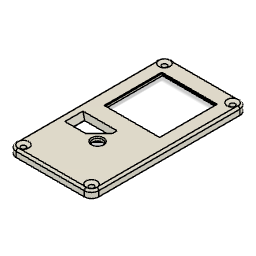
Marauder-Mini-Assembly (Autodesk Fusion 360 archive; units mm, degrees)
design "Marauder-Mini_Top_cutout"
Autodesk Fusion 360 part; units mm, degrees
sketch "Skizze1" plane through (0, 0, 0) normal (0, 1, 0) x (1, 0, 0)
  line L0 (1.75, 0) -> (22.5, 0)
  line L1 (0, -1.75) -> (0, -22.5)
  line L2 (-16.61, 36.93) -> (16.61, 36.93)
  line L3 (19.15, 34.39) -> (19.15, -34.39)
  line L4 (16.61, -36.93) -> (-16.61, -36.93)
  line L5 (-19.15, -34.39) -> (-19.15, 34.39)
  arc A0 (-16.61, 36.93) -> (-19.15, 34.39) centre (-16.61, 34.39) ccw
  arc A1 (19.15, 34.39) -> (16.61, 36.93) centre (16.61, 34.39) ccw
  arc A2 (16.61, -36.93) -> (19.15, -34.39) centre (16.61, -34.39) ccw
  arc A3 (-19.15, -34.39) -> (-16.61, -36.93) centre (-16.61, -34.39) ccw
  arc A4 (20.15, 34.39) -> (16.61, 37.93) centre (16.61, 34.39) ccw
  line L6 (-16.61, 37.93) -> (16.61, 37.93)
  arc A5 (-16.61, 37.93) -> (-20.15, 34.39) centre (-16.61, 34.39) ccw
  line L7 (-20.15, -34.39) -> (-20.15, 34.39)
  arc A6 (-20.15, -34.39) -> (-16.61, -37.93) centre (-16.61, -34.39) ccw
  line L8 (16.61, -37.93) -> (-16.61, -37.93)
  arc A7 (16.61, -37.93) -> (20.15, -34.39) centre (16.61, -34.39) ccw
  line L9 (20.15, 34.39) -> (20.15, -34.39)
  line L10 (-15.5, 32.25) -> (15.5, 32.25)
  line L11 (15.5, 32.25) -> (15.5, -4.75)
  line L12 (15.5, -4.75) -> (-15.5, -4.75)
  line L13 (-15.5, -4.75) -> (-15.5, 32.25)
  circle A8 centre (-16.61, 34.39) radius 1.2
  circle A9 centre (16.61, 34.39) radius 1.2
  circle A10 centre (-16.61, -34.39) radius 1.2
  circle A11 centre (16.61, -34.39) radius 1.2
  line L14 (-6.35, -27.43) -> (6.35, -27.43)
  line L15 (6.35, -27.43) -> (6.35, -35.43)
  line L16 (6.35, -35.43) -> (-6.35, -35.43)
  line L17 (-6.35, -35.43) -> (-6.35, -27.43)
  line L18 (-1.864, -10.43) -> (-4.5, -13.066)
  line L19 (-4.5, -13.066) -> (-4.5, -16.794)
  line L20 (-4.5, -16.794) -> (-1.864, -19.43)
  line L21 (-1.864, -19.43) -> (1.864, -19.43)
  line L22 (1.864, -19.43) -> (4.5, -16.794)
  line L23 (4.5, -16.794) -> (4.5, -13.066)
  line L24 (4.5, -13.066) -> (1.864, -10.43)
  line L25 (1.864, -10.43) -> (-1.864, -10.43)
  line L26 (0.5, -5.65) -> (15.5, -5.65)
  line L27 (15.5, -5.65) -> (15.5, -13.65)
  line L28 (15.5, -13.65) -> (6.5, -13.65)
  line L29 (6.5, -13.65) -> (0.5, -7.65)
  line L30 (0.5, -7.65) -> (0.5, -5.65)
  point P0 (-19.15, 36.93)
  point P1 (19.15, 36.93)
  point P2 (-19.15, -36.93)
  point P3 (0, -14.93)
  point P4 (0, -4.75)
  dimension "d1" = 73.86
  dimension "d2" = 38.3
  dimension "d3" = 2.54
  dimension "d4" = -1
  dimension "d5" = 31
  dimension "d7" = 2.4
  dimension "d8" = 37
  dimension "d9" = 8
  dimension "d10" = 12.7
  dimension "d11" = 1.5
  dimension "d12" = 22
  dimension "d24" = 4.5
  dimension "d27" = 8
  dimension "d28" = 15
  dimension "d30" = 2
  dimension "d47" = 5.65
  dimension "d48" = 4.75
  constraint horizontal L2
  constraint vertical L3
  constraint horizontal L4
  constraint vertical L5
  constraint symmetric L0 L2 L4
  constraint symmetric L1 L3 L5
  constraint coincident P0 L2
  constraint coincident P0 L5
  constraint tangent L2 A0
  constraint tangent L5 A0
  constraint coincident P1 L2
  constraint coincident P1 L3
  constraint tangent L2 A1
  constraint tangent L3 A1
  constraint equal A0 A1
  constraint tangent L3 A2
  constraint tangent L4 A2
  constraint equal A0 A2
  constraint coincident P2 L4
  constraint coincident P2 L5
  constraint tangent L4 A3
  constraint tangent L5 A3
  constraint equal A0 A3
  constraint horizontal L10
  constraint vertical L11
  constraint horizontal L12
  constraint vertical L13
  constraint symmetric L1 L11 L13
  constraint concentric A0 A8
  constraint concentric A1 A9
  constraint concentric A3 A10
  constraint concentric A2 A11
  constraint equal A10 A11
  constraint equal A9 A11
  constraint equal A8 A9
  constraint horizontal L14
  constraint vertical L15
  constraint horizontal L16
  constraint vertical L17
  constraint symmetric L1 L15 L17
  constraint horizontal L25
  constraint midpoint L12 P4
  constraint vertical P3 P4
  constraint horizontal L26
  constraint perpendicular L26 L27
  constraint perpendicular L27 L28
  constraint vertical L30
  constraint parallel L24 L29
  constraint collinear L11 L27
  constraint coincident L28.end L29.start
  measures "d1" distance of P0 P2
  measures "d2" distance of P0 P1
  measures "d3" radius of A0
  measures "d5" distance of L10.start L10.end
  measures "d7" diameter of A8
  measures "d8" distance of L10.end L11.end
  measures "d9" distance of L14.end L15.end
  measures "d10" distance of L15.end L16.end
  measures "d11" distance of L4 L16
  measures "d12" distance of L4 P3
  measures "d24" distance of P3 L25
  measures "d27" distance of L26.end L27.end
  measures "d28" distance of L26.start L26.end
  measures "d30" distance of L26.start L29.end
  measures "d47" distance of origin L26
  measures "d48" distance of origin L12
extrude "Extrusion1" add sketch "Skizze1" along normal blind 2 contours L2 L3 L4 L5 A0 A1 A2 A3 | A4 L6 A5 L7 A6 L8 A7 L9 makes body 1
sketch "Skizze2" plane through (0, 2, 0) normal (0, 1, 0) x (-1, 0, 0)
  circle A0 centre (16.61, -34.39) radius 1.2
  line L0 (-6.35, 35.43) -> (6.35, 35.43)
  line L1 (6.35, 35.43) -> (6.35, 27.43)
  line L2 (6.35, 27.43) -> (-6.35, 27.43)
  line L3 (-6.35, 27.43) -> (-6.35, 35.43)
  circle A1 centre (-16.61, 34.39) radius 1.2
  circle A2 centre (-16.61, -34.39) radius 1.2
  circle A3 centre (16.61, 34.39) radius 1.2
  line L4 (-15.5, 4.75) -> (15.5, 4.75)
  line L5 (15.5, 4.75) -> (15.5, -32.25)
  line L6 (15.5, -32.25) -> (-15.5, -32.25)
  line L7 (-15.5, -32.25) -> (-15.5, 4.75)
  arc A4 (16.61, -37.93) -> (20.15, -34.39) centre (16.61, -34.39) ccw
  line L8 (20.15, -34.39) -> (20.15, 34.39)
  arc A5 (20.15, 34.39) -> (16.61, 37.93) centre (16.61, 34.39) ccw
  line L9 (16.61, 37.93) -> (-16.61, 37.93)
  arc A6 (-16.61, 37.93) -> (-20.15, 34.39) centre (-16.61, 34.39) ccw
  line L10 (-20.15, 34.39) -> (-20.15, -34.39)
  arc A7 (-20.15, -34.39) -> (-16.61, -37.93) centre (-16.61, -34.39) ccw
  line L11 (-16.61, -37.93) -> (16.61, -37.93)
  circle A8 centre (0, 14.83) radius 2.5
  line L12 (1.864, 10.43) -> (-1.864, 10.43)
  line L13 (-1.864, 10.43) -> (-4.5, 13.066)
  line L14 (-4.5, 13.066) -> (-4.5, 16.794)
  line L15 (-4.5, 16.794) -> (-1.864, 19.43)
  line L16 (-1.864, 19.43) -> (1.864, 19.43)
  line L17 (1.864, 19.43) -> (4.5, 16.794)
  line L18 (4.5, 16.794) -> (4.5, 13.066)
  line L19 (4.5, 13.066) -> (1.864, 10.43)
  line L20 (-6.5, 13.65) -> (-0.5, 7.65)
  line L21 (-0.5, 7.65) -> (-0.5, 5.65)
  line L22 (-0.5, 5.65) -> (-15.5, 5.65)
  line L23 (-15.5, 5.65) -> (-15.5, 13.65)
  line L24 (-15.5, 13.65) -> (-6.5, 13.65)
  dimension "d16" = 5
  measures "d16" diameter of A8
extrude "Extrusion2" add sketch "Skizze2" along normal blind 1 contours L0 L1 L2 L3 | A4 L8 A5 L9 A6 L10 A7 L11 | L12 L13 L14 L15 L16 L17 L18 L19 bodies 1
chamfer "Fase4" distance 0.5 distance2 1 8 edges at (4.5, 2, 14.93) (3.182, 2, 18.112) (0, 2, 19.43) (-3.182, 2, 18.112) (-4.5, 2, 14.93) (-3.182, 2, 11.748) (3.182, 2, 11.748) (0, 2, 10.43) measured on face at (0.0623, 2, 18.7277) measured on face at (0.0623, 2, 18.7277) measured on face at (0.0623, 2, 18.7277) measured on face at (0.0623, 2, 18.7277) measured on face at (0.0623, 2, 18.7277) measured on face at (0.0623, 2, 18.7277) measured on face at (0.0623, 2, 18.7277) measured on face at (0.0623, 2, 18.7277) on bodies 1
sketch "Skizze3" plane through (0, 3, 0) normal (0, 1, 0) x (-1, 0, 0)
  circle A0 centre (0, 14.83) radius 2.5
  circle A1 centre (-16.61, -34.39) radius 1.2
  circle A2 centre (16.61, -34.39) radius 1.2
  line L0 (15.5, -32.25) -> (-15.5, -32.25)
  line L1 (-15.5, -32.25) -> (-15.5, 4.75)
  line L2 (-15.5, 4.75) -> (15.5, 4.75)
  line L3 (15.5, 4.75) -> (15.5, -32.25)
  circle A3 centre (-16.61, 34.39) radius 1.2
  line L4 (-15.5, 5.65) -> (-15.5, 13.65)
  line L5 (-15.5, 13.65) -> (-6.5, 13.65)
  line L6 (-6.5, 13.65) -> (-0.5, 7.65)
  line L7 (-0.5, 7.65) -> (-0.5, 5.65)
  line L8 (-0.5, 5.65) -> (-15.5, 5.65)
  circle A4 centre (16.61, 34.39) radius 1.2
  line L9 (-16.61, -37.93) -> (16.61, -37.93)
  arc A5 (16.61, -37.93) -> (20.15, -34.39) centre (16.61, -34.39) ccw
  line L10 (20.15, -34.39) -> (20.15, 34.39)
  arc A6 (20.15, 34.39) -> (16.61, 37.93) centre (16.61, 34.39) ccw
  line L11 (16.61, 37.93) -> (-16.61, 37.93)
  arc A7 (-16.61, 37.93) -> (-20.15, 34.39) centre (-16.61, 34.39) ccw
  line L12 (-20.15, 34.39) -> (-20.15, -34.39)
  arc A8 (-20.15, -34.39) -> (-16.61, -37.93) centre (-16.61, -34.39) ccw
  line L13 (0, 1.75) -> (0, 22.5)
  line L14 (13.5, -29.93) -> (-13.5, -29.93)
  line L15 (-13.5, -29.93) -> (-13.5, -1.93)
  line L16 (-13.5, -1.93) -> (13.5, -1.93)
  line L17 (13.5, -1.93) -> (13.5, -29.93)
  dimension "d33" = 27
  dimension "d49" = 28
  dimension "d50" = 8
  constraint horizontal L14
  constraint vertical L15
  constraint horizontal L16
  constraint vertical L17
  constraint symmetric L13 L15 L17
  measures "d33" distance of L15 L17
  measures "d49" distance of L14 L16
  measures "d50" distance of L9 L14
extrude "Extrusion3" add sketch "Skizze3" along normal blind 0.6 contours L0 L1 L2 L3 | L9 A5 L10 A6 L11 A7 L12 A8 bodies 1
fillet "Abrundung2" radius 1 8 edges at (0, 3.6, 37.93) (19.1132, 3.6, 36.8932) (20.15, 3.6, 0) (19.1132, 3.6, -36.8932) (0, 3.6, -37.93) (-19.1132, 3.6, -36.8932) (-20.15, 3.6, 0) (-19.1132, 3.6, 36.8932) on bodies 1
chamfer "Fase5" distance 1.5 distance2 1 4 edges at (-15.4912, 3.6, -33.9561) (17.7288, 3.6, -33.9561) (17.7288, 3.6, 34.8239) (-15.4912, 3.6, 34.8239) measured on face at (0, 3.6, 28.5841) measured on face at (0, 3.6, 28.5841) measured on face at (0, 3.6, 28.5841) measured on face at (0, 3.6, 28.5841) on bodies 1
chamfer "Fase6" distance 0.5 distance2 0.5 1 edges at (2.3308, 3.6, 15.734) measured on face at (-0.0585, 3.6, 28.4655) on bodies 1
chamfer "Fase6" distance 2 angle 45 4 edges at (0, 2, 27.43) (-6.35, 2, 31.43) (0, 2, 35.43) (6.35, 2, 31.43) on bodies 1
chamfer "Fase7" distance 0.8 distance2 3.5 4 edges at (0.5, 3.6, 6.65) (3.5, 3.6, 10.65) (11, 3.6, 13.65) (15.5, 3.6, 9.65) measured on face at (-0.071, 3.6, 28.6317) measured on face at (-0.071, 3.6, 28.6317) measured on face at (-0.071, 3.6, 28.6317) measured on face at (-0.071, 3.6, 28.6317) on bodies 1
mirror "Spiegeln1" about plane through (20.15, 3, 34.39) normal (1, 0, 0) of bodies 1 makes body 2
hidden bodies 1
equation "d5 = 30.1 mm + 0.9 mm"
named bodies: "MarauderMini-Top"

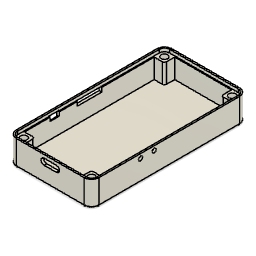
design "Marauder-Mini_Bottom"
Autodesk Fusion 360 part; units mm, degrees
sketch "Skizze1" plane through (0, 0, 0) normal (0, 1, 0) x (1, 0, 0)
  line L0 (-16.51, 36.83) -> (16.51, 36.83)
  line L1 (19.05, 34.29) -> (19.05, -34.29)
  line L2 (16.51, -36.83) -> (-16.51, -36.83)
  line L3 (-19.05, -34.29) -> (-19.05, 34.29)
  line L4 (1.75, 0) -> (22.5, 0)
  line L5 (0, -1.75) -> (0, -22.5)
  arc A0 (-16.51, 36.83) -> (-19.05, 34.29) centre (-16.51, 34.29) ccw
  arc A1 (19.05, 34.29) -> (16.51, 36.83) centre (16.51, 34.29) ccw
  arc A2 (16.51, -36.83) -> (19.05, -34.29) centre (16.51, -34.29) ccw
  arc A3 (-19.05, -34.29) -> (-16.51, -36.83) centre (-16.51, -34.29) ccw
  arc A4 (20.15, 34.29) -> (16.51, 37.93) centre (16.51, 34.29) ccw
  line L6 (-16.51, 37.93) -> (16.51, 37.93)
  arc A5 (-16.51, 37.93) -> (-20.15, 34.29) centre (-16.51, 34.29) ccw
  line L7 (-20.15, -34.29) -> (-20.15, 34.29)
  arc A6 (-20.15, -34.29) -> (-16.51, -37.93) centre (-16.51, -34.29) ccw
  line L8 (16.51, -37.93) -> (-16.51, -37.93)
  arc A7 (16.51, -37.93) -> (20.15, -34.29) centre (16.51, -34.29) ccw
  line L9 (20.15, 34.29) -> (20.15, -34.29)
  point P0 (-19.05, 36.83)
  point P1 (19.05, 36.83)
  point P2 (-19.05, -36.83)
  dimension "d1" = 73.66
  dimension "d2" = 38.1
  dimension "d3" = 2.54
  dimension "d4" = -1.1
  constraint horizontal L0
  constraint vertical L1
  constraint horizontal L2
  constraint vertical L3
  constraint symmetric L0 L2 L4
  constraint symmetric L1 L3 L5
  constraint coincident P0 L0
  constraint coincident P0 L3
  constraint tangent L0 A0
  constraint tangent L3 A0
  constraint coincident P1 L0
  constraint coincident P1 L1
  constraint tangent L0 A1
  constraint tangent L1 A1
  constraint equal A0 A1
  constraint tangent L1 A2
  constraint tangent L2 A2
  constraint equal A0 A2
  constraint coincident P2 L2
  constraint coincident P2 L3
  constraint tangent L2 A3
  constraint tangent L3 A3
  constraint equal A0 A3
  measures "d1" distance of P0 P2
  measures "d2" distance of P0 P1
  measures "d3" radius of A0
extrude "Extrusion1" add sketch "Skizze1" along normal blind 1.5 contours L0 L1 L2 L3 A0 A1 A2 A3 | A4 L6 A5 L7 A6 L8 A7 L9
sketch "Skizze2" plane through (0, 1.5, 0) normal (0, 1, 0) x (-1, 0, 0)
  arc A0 (16.51, -37.93) -> (20.15, -34.29) centre (16.51, -34.29) ccw
  line L0 (20.15, -34.29) -> (20.15, 34.29)
  arc A1 (20.15, 34.29) -> (16.51, 37.93) centre (16.51, 34.29) ccw
  line L1 (16.51, 37.93) -> (-16.51, 37.93)
  arc A2 (-16.51, 37.93) -> (-20.15, 34.29) centre (-16.51, 34.29) ccw
  line L2 (-20.15, 34.29) -> (-20.15, -34.29)
  arc A3 (-20.15, -34.29) -> (-16.51, -37.93) centre (-16.51, -34.29) ccw
  line L3 (-16.51, -37.93) -> (16.51, -37.93)
  line L4 (18.85, -34.29) -> (18.85, 34.29)
  arc A4 (18.85, 34.29) -> (16.51, 36.63) centre (16.51, 34.29) ccw
  line L5 (16.51, 36.63) -> (-16.51, 36.63)
  arc A5 (-16.51, 36.63) -> (-18.85, 34.29) centre (-16.51, 34.29) ccw
  line L6 (-18.85, 34.29) -> (-18.85, -34.29)
  arc A6 (-18.85, -34.29) -> (-16.51, -36.63) centre (-16.51, -34.29) ccw
  line L7 (-16.51, -36.63) -> (16.51, -36.63)
  arc A7 (16.51, -36.63) -> (18.85, -34.29) centre (16.51, -34.29) ccw
  circle A8 centre (16.51, -34.29) radius 1.65
  circle A9 centre (-16.51, -34.29) radius 1.65
  circle A10 centre (-16.51, 34.29) radius 1.65
  circle A11 centre (16.51, 34.29) radius 1.65
  line L8 (13.85, -36.63) -> (13.85, -32.63)
  line L9 (14.85, -31.63) -> (18.85, -31.63)
  line L10 (-13.85, -36.63) -> (-13.85, -32.63)
  line L11 (-14.85, -31.63) -> (-18.85, -31.63)
  line L12 (18.85, 31.63) -> (14.85, 31.63)
  line L13 (13.85, 32.63) -> (13.85, 36.63)
  line L14 (-13.85, 36.63) -> (-13.85, 32.63)
  line L15 (-14.85, 31.63) -> (-18.85, 31.63)
  line L16 (-1.75, 0) -> (-22.5, 0)
  line L17 (0, 1.75) -> (0, 22.5)
  arc A12 (14.85, -31.63) -> (13.85, -32.63) centre (14.85, -32.63) ccw
  arc A13 (-13.85, -32.63) -> (-14.85, -31.63) centre (-14.85, -32.63) ccw
  arc A14 (13.85, 32.63) -> (14.85, 31.63) centre (14.85, 32.63) ccw
  arc A15 (-14.85, 31.63) -> (-13.85, 32.63) centre (-14.85, 32.63) ccw
  point P0 (13.85, -31.63)
  dimension "d7" = -1.3
  dimension "d8" = 3.3
  dimension "d9" = 5
  dimension "d10" = 5
  dimension "d11" = 1
  constraint concentric A0 A8
  constraint concentric A3 A9
  constraint concentric A2 A10
  constraint concentric A1 A11
  constraint equal A8 A9
  constraint equal A9 A10
  constraint equal A10 A11
  constraint coincident L7 L8.start
  constraint perpendicular L7 L8
  constraint coincident L4 L9.end
  constraint perpendicular L4 L9
  constraint coincident L7 L10.start
  constraint perpendicular L7 L10
  constraint perpendicular L10 L11
  constraint coincident L4 L12.start
  constraint perpendicular L4 L12
  constraint coincident L5 L13.end
  constraint perpendicular L5 L13
  constraint coincident L5 L14.start
  constraint perpendicular L5 L14
  constraint perpendicular L14 L15
  constraint collinear L9 L11
  constraint collinear L8 L13
  constraint collinear L12 L15
  constraint collinear L10 L14
  constraint symmetric L9 L12 L16
  constraint symmetric L8 L10 L17
  constraint coincident P0 L8
  constraint coincident P0 L9
  constraint tangent L8 A12
  constraint tangent L9 A12
  constraint tangent L10 A13
  constraint tangent L11 A13
  constraint equal A12 A13
  constraint tangent L12 A14
  constraint tangent L13 A14
  constraint equal A12 A14
  constraint tangent L14 A15
  constraint tangent L15 A15
  constraint equal A12 A15
  constraint coincident L6 L11.end
  constraint coincident L6 L15.end
  measures "d8" diameter of A8
  measures "d9" distance of L8.start P0
  measures "d10" distance of P0 L9.end
  measures "d11" radius of A12
extrude "Extrusion2" add sketch "Skizze2" along normal blind 9.5 contours A0 L0 A1 L1 A2 L2 A3 L3 | L4 L7 A7 L8 L9 A12 | L4 A4 L5 L12 L13 A14 | L6 A6 L7 L10 L11 A13 | L5 A5 L6 L14 L15 A15
fillet "Abrundung1" radius 1 8 edges at (-19.0839, 0, -36.8639) (0, 0, -37.93) (19.0839, 0, -36.8639) (20.15, 0, 0) (19.0839, 0, 36.8639) (0, 0, 37.93) (-19.0839, 0, 36.8639) (-20.15, 0, 0)
sketch "Skizze3" plane through (0, 0, 37.93) normal (0, 0, 1) x (1, 0, 0)
  line L0 (-16.51, 1) -> (16.51, 1)
  line L1 (16.51, 1) -> (16.51, 11)
  line L2 (16.51, 11) -> (-16.51, 11)
  line L3 (-16.51, 11) -> (-16.51, 1)
  line L4 (-4.5, 11) -> (4.5, 11)
  line L5 (4.5, 11) -> (4.5, 8)
  line L6 (4.5, 8) -> (-4.5, 8)
  line L7 (-4.5, 8) -> (-4.5, 11)
  line L8 (0, 1.75) -> (0, 22.5)
  dimension "d16" = 9
  dimension "d17" = 3
  constraint horizontal L4
  constraint vertical L5
  constraint horizontal L6
  constraint vertical L7
  constraint coincident L2 L4.start
  constraint symmetric L5 L7 L8
  measures "d16" distance of L5.end L6.end
  measures "d17" distance of L4.start L6.end
extrude "Extrusion3" cut sketch "Skizze3" against normal blind 2 contours L2 L4 L6 L7 L8 | L2 L4 L5 L6 L8
sketch "Skizze4" plane through (-20.15, 0, 0) normal (-1, 0, 0) x (0, 0, 1)
  line L0 (-34.29, 1) -> (34.29, 1)
  line L1 (34.29, 11) -> (-34.29, 11)
  line L2 (-34.29, 11) -> (-34.29, 1)
  line L3 (14.63, 11) -> (19.13, 11)
  line L4 (19.13, 11) -> (19.13, 9.2)
  line L5 (19.13, 9.2) -> (14.63, 9.2)
  line L6 (14.63, 9.2) -> (14.63, 11)
  line L7 (-6.07, 11) -> (5.93, 11)
  line L8 (5.93, 11) -> (5.93, 9)
  line L9 (5.93, 9) -> (-6.07, 9)
  line L10 (-6.07, 9) -> (-6.07, 11)
  line L11 (36.63, 11) -> (36.63, 8)
  line L12 (36.63, 8) -> (36.63, 11)
  line L13 (36.63, 11) -> (36.63, 1.5)
  line L14 (36.63, 1.5) -> (36.63, 11)
  line L15 (37.93, 1) -> (37.93, 11)
  dimension "d22" = 4.5
  dimension "d23" = 1.8
  dimension "d24" = 17.5
  dimension "d25" = 12
  dimension "d26" = 2
  dimension "d56" = 32
  constraint horizontal L3
  constraint vertical L4
  constraint horizontal L5
  constraint vertical L6
  constraint coincident L1 L3.start
  constraint horizontal L7
  constraint vertical L8
  constraint horizontal L9
  constraint vertical L10
  constraint coincident L1 L7.start
  measures "d22" distance of L4.end L5.end
  measures "d23" distance of L3.end L4.end
  measures "d24" distance of L4 L13
  measures "d25" distance of L8.end L9.end
  measures "d26" distance of L7.start L9.end
  measures "d56" distance of L8 L15
extrude "Extrusion4" cut sketch "Skizze4" against normal blind 2
sketch "Skizze6" plane through (0, 11, 0) normal (0, 1, 0) x (-1, 0, 0)
  line L0 (-16.51, -37.93) -> (16.51, -37.93)
  arc A0 (16.51, -37.93) -> (20.15, -34.29) centre (16.51, -34.29) ccw
  line L1 (20.15, -34.29) -> (20.15, -6.07)
  line L2 (20.15, -6.07) -> (18.85, -6.07)
  line L3 (18.85, -6.07) -> (18.85, -31.63)
  line L4 (18.85, -31.63) -> (14.85, -31.63)
  arc A1 (14.85, -31.63) -> (13.85, -32.63) centre (14.85, -32.63) ccw
  line L5 (13.85, -32.63) -> (13.85, -36.63)
  line L6 (13.85, -36.63) -> (-13.85, -36.63)
  circle A2 centre (16.51, -34.29) radius 1.65
  line L7 (13.85, -36.63) -> (-13.85, -36.63)
  line L8 (-13.85, -36.63) -> (-13.85, -32.63)
  arc A3 (-13.85, -32.63) -> (-14.85, -31.63) centre (-14.85, -32.63) ccw
  line L9 (-14.85, -31.63) -> (-18.85, -31.63)
  line L10 (-18.85, -31.63) -> (-18.85, 31.63)
  line L11 (-18.85, 31.63) -> (-14.85, 31.63)
  arc A4 (-14.85, 31.63) -> (-13.85, 32.63) centre (-14.85, 32.63) ccw
  line L12 (-13.85, 32.63) -> (-13.85, 36.63)
  line L13 (-13.85, 36.63) -> (-4.5, 36.63)
  line L14 (-4.5, 36.63) -> (-4.5, 37.93)
  line L15 (-4.5, 37.93) -> (-16.51, 37.93)
  arc A5 (-16.51, 37.93) -> (-20.15, 34.29) centre (-16.51, 34.29) ccw
  line L16 (-20.15, 34.29) -> (-20.15, -34.29)
  arc A6 (-20.15, -34.29) -> (-16.51, -37.93) centre (-16.51, -34.29) ccw
  line L17 (-16.51, -37.93) -> (16.51, -37.93)
  circle A7 centre (-16.51, 34.29) radius 1.65
  circle A8 centre (-16.51, -34.29) radius 1.65
  line L18 (18.85, 19.13) -> (20.15, 19.13)
  line L19 (20.15, 19.13) -> (20.15, 34.29)
  arc A9 (20.15, 34.29) -> (16.51, 37.93) centre (16.51, 34.29) ccw
  line L20 (16.51, 37.93) -> (4.5, 37.93)
  line L21 (4.5, 37.93) -> (4.5, 36.63)
  line L22 (4.5, 36.63) -> (13.85, 36.63)
  line L23 (13.85, 36.63) -> (13.85, 32.63)
  arc A10 (13.85, 32.63) -> (14.85, 31.63) centre (14.85, 32.63) ccw
  line L24 (14.85, 31.63) -> (18.85, 31.63)
  line L25 (18.85, 31.63) -> (18.85, 19.13)
  circle A11 centre (16.51, 34.29) radius 1.65
  line L26 (16.81, -37.13) -> (-16.81, -37.13)
  line L27 (-19.35, 34.59) -> (-19.35, -34.59)
  line L28 (18.85, 5.93) -> (20.15, 5.93)
  line L29 (20.15, 5.93) -> (20.15, 14.63)
  line L30 (20.15, 14.63) -> (18.85, 14.63)
  line L31 (18.85, 14.63) -> (18.85, 5.93)
  line L32 (20.15, 19.13) -> (20.15, 14.63)
  line L33 (20.15, 5.93) -> (20.15, -6.07)
  line L34 (-13.85, -36.63) -> (-13.85, -32.63)
  arc A12 (-13.85, -32.63) -> (-14.85, -31.63) centre (-14.85, -32.63) ccw
  line L35 (-14.85, -31.63) -> (-18.85, -31.63)
  line L36 (-18.85, -31.63) -> (-18.85, 31.63)
  line L37 (-18.85, 31.63) -> (-14.85, 31.63)
  arc A13 (-14.85, 31.63) -> (-13.85, 32.63) centre (-14.85, 32.63) ccw
  line L38 (-13.85, 32.63) -> (-13.85, 36.63)
  line L39 (-13.85, 36.63) -> (-4.5, 36.63)
  line L40 (-4.5, 36.63) -> (-4.5, 37.93)
  line L41 (-4.5, 37.93) -> (-16.51, 37.93)
  arc A14 (-16.51, 37.93) -> (-20.15, 34.29) centre (-16.51, 34.29) ccw
  line L42 (-20.15, 34.29) -> (-20.15, -34.29)
  arc A15 (-20.15, -34.29) -> (-16.51, -37.93) centre (-16.51, -34.29) ccw
  circle A16 centre (-16.51, 34.29) radius 1.65
  circle A17 centre (-16.51, -34.29) radius 1.65
  line L43 (20.15, -6.07) -> (18.85, -6.07)
  line L44 (18.85, -6.07) -> (18.85, -31.63)
  line L45 (18.85, -31.63) -> (14.85, -31.63)
  arc A18 (14.85, -31.63) -> (13.85, -32.63) centre (14.85, -32.63) ccw
  line L46 (13.85, -32.63) -> (13.85, -36.63)
  arc A19 (16.51, -37.93) -> (20.15, -34.29) centre (16.51, -34.29) ccw
  line L47 (20.15, -34.29) -> (20.15, -6.07)
  circle A20 centre (16.51, -34.29) radius 1.65
  line L48 (4.5, 37.93) -> (-4.5, 37.93)
  line L49 (16.81, 37.13) -> (14.85, 37.13)
  line L50 (14.85, 37.13) -> (-16.81, 37.13)
  line L51 (19.35, 34.59) -> (19.35, -34.59)
  arc A21 (-16.81, 37.13) -> (-19.35, 34.59) centre (-16.81, 34.59) ccw
  arc A22 (19.35, 34.59) -> (16.81, 37.13) centre (16.81, 34.59) ccw
  arc A23 (16.81, -37.13) -> (19.35, -34.59) centre (16.81, -34.59) ccw
  arc A24 (-19.35, -34.59) -> (-16.81, -37.13) centre (-16.81, -34.59) ccw
  dimension "d52" = 0.8
  dimension "d53" = 0.8
  dimension "d54" = 2.54
  constraint coincident L20.end L21.start
  constraint coincident L14.end L15.start
  constraint vertical L51
  constraint horizontal L26
  constraint horizontal L50
  constraint vertical L27
  constraint tangent L50 A21
  constraint tangent L49 A22
  constraint tangent L51 A23
  constraint tangent L26 A24
  constraint equal A23 A24
  constraint equal A22 A23
  constraint equal A21 A22
  constraint tangent L27 A21
  constraint tangent L51 A22
  constraint coincident L26.start A23.start
  constraint tangent L26 A23
  constraint tangent L27 A24
  measures "d52" distance of L19 L51
  measures "d53" distance of L27 L42
  measures "d54" radius of A21
extrude "Extrusion6" add sketch "Skizze6" along normal blind 1.55 contours L0 A0 L1 L2 L14 L15 A5 L16 A6 L17 L26 L27 L40 L41 A14 L42 A15 L43 A19 L47 L50 L51 A21 A23 A24 | L2 L28 L33 L43 L51 | L28 L29 L30 L51 | L14 L21 L40 L48 L50 | L18 L30 L32 L51 | L18 L19 A9 L20 L21 L49 L50 L51 A22
sketch "Skizze7" plane through (20.15, 0, 0) normal (1, 0, 0) x (0, 0, -1)
  line L0 (-34.29, 1) -> (34.29, 1)
  line L1 (34.29, 1) -> (34.29, 12.55)
  line L2 (34.29, 12.55) -> (-34.29, 12.55)
  line L3 (-34.29, 12.55) -> (-34.29, 1)
  circle A0 centre (-14.03, 10.5) radius 1
  circle A1 centre (-7.42, 10.5) radius 1
  line L4 (-36.63, 11) -> (-36.63, 8)
  line L5 (-36.63, 8) -> (-36.63, 11)
  line L6 (-36.63, 11) -> (-36.63, 1.5)
  line L7 (-36.63, 1.5) -> (-36.63, 11)
  dimension "d42" = 2
  dimension "d43" = 22.6
  dimension "d44" = 29.21
  dimension "d45" = 9.5
  constraint equal A0 A1
  constraint horizontal A0.centre A1.centre
  measures "d42" diameter of A0
  measures "d43" distance of A0.centre L6
  measures "d44" distance of A1.centre L4
  measures "d45" distance of L0 A0.centre
extrude "Extrusion7" cut sketch "Skizze7" against normal blind 3 contours A0 | A1
extrude "Extrusion8" cut 1 faces at (-19.6167, 11, 16.13) along direction (0, 1, 0) blind 0.2
fillet "Fillet2" radius 1.5 4 edges at (4.5, 8, 37.28) (4.5, 11, 37.53) (-4.5, 11, 37.53) (-4.5, 8, 37.28)
chamfer "Chamfer1" distance 0.8 angle 45 2 edges at (-20.15, 11.2, 16.88) (-20.15, 9.2, 16.88)
named bodies: "MarauderMini-Bottom"

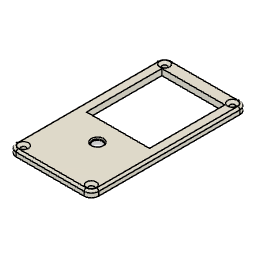
design "Marauder-Mini_Top"
Autodesk Fusion 360 part; units mm, degrees
sketch "Skizze1" plane through (0, 0, 0) normal (0, 1, 0) x (1, 0, 0)
  line L0 (1.75, 0) -> (22.5, 0)
  line L1 (0, -1.75) -> (0, -22.5)
  line L2 (-16.51, 36.83) -> (16.51, 36.83)
  line L3 (19.05, 34.29) -> (19.05, -34.29)
  line L4 (16.51, -36.83) -> (-16.51, -36.83)
  line L5 (-19.05, -34.29) -> (-19.05, 34.29)
  arc A0 (-16.51, 36.83) -> (-19.05, 34.29) centre (-16.51, 34.29) ccw
  arc A1 (19.05, 34.29) -> (16.51, 36.83) centre (16.51, 34.29) ccw
  arc A2 (16.51, -36.83) -> (19.05, -34.29) centre (16.51, -34.29) ccw
  arc A3 (-19.05, -34.29) -> (-16.51, -36.83) centre (-16.51, -34.29) ccw
  arc A4 (20.05, 34.29) -> (16.51, 37.83) centre (16.51, 34.29) ccw
  line L6 (-16.51, 37.83) -> (16.51, 37.83)
  arc A5 (-16.51, 37.83) -> (-20.05, 34.29) centre (-16.51, 34.29) ccw
  line L7 (-20.05, -34.29) -> (-20.05, 34.29)
  arc A6 (-20.05, -34.29) -> (-16.51, -37.83) centre (-16.51, -34.29) ccw
  line L8 (16.51, -37.83) -> (-16.51, -37.83)
  arc A7 (16.51, -37.83) -> (20.05, -34.29) centre (16.51, -34.29) ccw
  line L9 (20.05, 34.29) -> (20.05, -34.29)
  line L10 (-15.3, 31.75) -> (15.3, 31.75)
  line L11 (15.3, 31.75) -> (15.3, -4.85)
  line L12 (15.3, -4.85) -> (-15.3, -4.85)
  line L13 (-15.3, -4.85) -> (-15.3, 31.75)
  circle A8 centre (-16.51, 34.29) radius 1.2
  circle A9 centre (16.51, 34.29) radius 1.2
  circle A10 centre (-16.51, -34.29) radius 1.2
  circle A11 centre (16.51, -34.29) radius 1.2
  circle A12 centre (0, -14.83) radius 6.5
  line L14 (-6.35, -27.33) -> (6.35, -27.33)
  line L15 (6.35, -27.33) -> (6.35, -35.33)
  line L16 (6.35, -35.33) -> (-6.35, -35.33)
  line L17 (-6.35, -35.33) -> (-6.35, -27.33)
  point P0 (-19.05, 36.83)
  point P1 (19.05, 36.83)
  point P2 (-19.05, -36.83)
  dimension "d1" = 73.66
  dimension "d2" = 38.1
  dimension "d3" = 2.54
  dimension "d4" = -1
  dimension "d5" = 30.6
  dimension "d6" = 5.08
  dimension "d7" = 2.4
  dimension "d8" = 36.6
  dimension "d9" = 8
  dimension "d10" = 12.7
  dimension "d11" = 1.5
  dimension "d12" = 22
  dimension "d13" = 13
  constraint horizontal L2
  constraint vertical L3
  constraint horizontal L4
  constraint vertical L5
  constraint symmetric L0 L2 L4
  constraint coincident P0 L2
  constraint coincident P0 L5
  constraint tangent L2 A0
  constraint tangent L5 A0
  constraint coincident P1 L2
  constraint coincident P1 L3
  constraint tangent L2 A1
  constraint tangent L3 A1
  constraint equal A0 A1
  constraint tangent L3 A2
  constraint tangent L4 A2
  constraint equal A0 A2
  constraint coincident P2 L4
  constraint coincident P2 L5
  constraint tangent L4 A3
  constraint tangent L5 A3
  constraint equal A0 A3
  constraint horizontal L10
  constraint vertical L11
  constraint horizontal L12
  constraint vertical L13
  constraint symmetric L1 L11 L13
  constraint concentric A0 A8
  constraint concentric A1 A9
  constraint concentric A3 A10
  constraint concentric A2 A11
  constraint equal A10 A11
  constraint equal A9 A11
  constraint equal A8 A9
  constraint coincident L1 A12.centre
  constraint horizontal L14
  constraint vertical L15
  constraint horizontal L16
  constraint vertical L17
  constraint symmetric L1 L15 L17
  measures "d1" distance of P0 P2
  measures "d2" distance of P0 P1
  measures "d3" radius of A0
  measures "d5" distance of L10.start L10.end
  measures "d6" distance of L2 L10
  measures "d7" diameter of A8
  measures "d8" distance of L10.end L11.end
  measures "d9" distance of L14.end L15.end
  measures "d10" distance of L15.end L16.end
  measures "d11" distance of L4 L16
  measures "d12" distance of L4 A12.centre
  measures "d13" diameter of A12
extrude "Extrusion1" add sketch "Skizze1" along normal blind 2 contours L2 L3 L4 L5 A0 A1 A2 A3 | A4 L6 A5 L7 A6 L8 A7 L9
sketch "Skizze2" plane through (0, 2, 0) normal (0, 1, 0) x (-1, 0, 0)
  circle A0 centre (16.51, -34.29) radius 1.2
  line L0 (-6.35, 35.33) -> (6.35, 35.33)
  line L1 (6.35, 35.33) -> (6.35, 27.33)
  line L2 (6.35, 27.33) -> (-6.35, 27.33)
  line L3 (-6.35, 27.33) -> (-6.35, 35.33)
  circle A1 centre (-16.51, 34.29) radius 1.2
  circle A2 centre (-16.51, -34.29) radius 1.2
  circle A3 centre (16.51, 34.29) radius 1.2
  line L4 (-15.3, 4.85) -> (15.3, 4.85)
  line L5 (15.3, 4.85) -> (15.3, -31.75)
  line L6 (15.3, -31.75) -> (-15.3, -31.75)
  line L7 (-15.3, -31.75) -> (-15.3, 4.85)
  circle A4 centre (0, 14.83) radius 6.5
  arc A5 (16.51, -37.83) -> (20.05, -34.29) centre (16.51, -34.29) ccw
  line L8 (20.05, -34.29) -> (20.05, 34.29)
  arc A6 (20.05, 34.29) -> (16.51, 37.83) centre (16.51, 34.29) ccw
  line L9 (16.51, 37.83) -> (-16.51, 37.83)
  arc A7 (-16.51, 37.83) -> (-20.05, 34.29) centre (-16.51, 34.29) ccw
  line L10 (-20.05, 34.29) -> (-20.05, -34.29)
  arc A8 (-20.05, -34.29) -> (-16.51, -37.83) centre (-16.51, -34.29) ccw
  line L11 (-16.51, -37.83) -> (16.51, -37.83)
  circle A9 centre (0, 14.83) radius 2.5
  dimension "d16" = 5
  constraint concentric A4 A9
  measures "d16" diameter of A9
extrude "Extrusion2" add sketch "Skizze2" along normal blind 1 contours L0 L1 L2 L3 | A4 | A5 L8 A6 L9 A7 L10 A8 L11
fillet "Abrundung1" radius 1 8 edges at (0, 3, 37.83) (19.0132, 3, 36.7932) (20.05, 3, 0) (19.0132, 3, -36.7932) (0, 3, -37.83) (-19.0132, 3, -36.7932) (-20.05, 3, 0) (-19.0132, 3, 36.7932)
chamfer "Fase1" distance 1.2 angle 45 4 edges at (-15.3912, 3, 34.7239) (17.6288, 3, 34.7239) (-15.3912, 3, -33.8561) (17.6288, 3, -33.8561)
chamfer "Fase2" distance 1 angle 45 1 edges at (-6.0601, 2, 12.4795)
chamfer "Fase3" distance 0.5 angle 45 1 edges at (2.3308, 3, 15.734)
equation "d5 = 30.1 mm + 0.5 mm"
equation "d6 = ( 2.54 * 2 ) * 1 mm"
